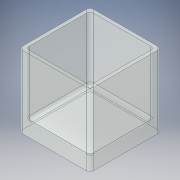
# Autodesk Inventor part: CandleHolder-3
Saved by Autodesk Inventor 2017 (Build 210142000, 142)
## iProperties
Created: 2016-10-20
Part Number: CandleHolder-3
Material: Glass
Document SubType Name: Modeling
Designer: Andrew Miyaguchi
Density: 2.18 g/cm^3
Appearance: Clear
Project: CandleHolder
Description: Glass Vase
Engineer: Andrew Miyaguchi
Author: andrew
Title: Glass Vase
Revision Number: 1
Autodesk Inventor part; units mm, degrees
ref_plane "YZ Plane" through (0, 0, 0) normal (1, 0, 0) x (0, 1, 0)
ref_plane "XZ Plane" through (0, 0, 0) normal (0, 1, 0) x (-1, 0, 0)
ref_plane "XY Plane" through (0, 0, 0) normal (0, 0, 1) x (1, 0, 0)
sketch "Sketch1" plane through (0, 0, 0) normal (0, 1, 0) x (-1, 0, 0)
  line L0 (-39.6875, 39.6875) -> (39.6875, 39.6875)
  line L1 (39.6875, 39.6875) -> (39.6875, -39.6875)
  line L2 (39.6875, -39.6875) -> (-39.6875, -39.6875)
  line L3 (-39.6875, -39.6875) -> (-39.6875, 39.6875)
  line L4 (-39.6875, 39.6875) -> (39.6875, -39.6875) construction
  line L5 (39.6875, 39.6875) -> (-39.6875, -39.6875) construction
  line L6 (-35.8775, 35.8775) -> (35.8775, 35.8775)
  line L7 (35.8775, 35.8775) -> (35.8775, -35.8775)
  line L8 (35.8775, -35.8775) -> (-35.8775, -35.8775)
  line L9 (-35.8775, -35.8775) -> (-35.8775, 35.8775)
  line L10 (-35.8775, 35.8775) -> (35.8775, -35.8775) construction
  line L11 (35.8775, 35.8775) -> (-35.8775, -35.8775) construction
  line L12 (0, -55.5625) -> (0, 55.5625) projected
  point P0 (0, 0)
  dimension "d0" = 3.81
  dimension "d10" = 79.375
  dimension "d11" = 45
  constraints: 24 end point, 4 midpoint, 4 parallel, 2 horizontal, 2 perpendicular, 1 point on line
  measures "d0" distance between parallel lines of L1 L7
  measures "d10" distance of L0.end L1.end
  measures "d11" angle of L12 L5
extrude "Extrusion1" add sketch "Sketch1" along normal blind 80.772 contours L0 L12 L6 L9 L8 L2 L3 | L0 L1 L2 L12 L8 L7 L6
extrude "Extrusion2" add sketch "Sketch1" along normal blind 9.652 contours L12 L8 L9 L6 | L6 L7 L8 L12
fillet "Fillet1" radius 3.81 12 edges at (-39.6875, 40.386, 39.6875) (-35.8775, 45.212, 35.8775) (-39.6875, 40.386, -39.6875) (-35.8775, 45.212, -35.8775) (35.8775, 45.212, -35.8775) (39.6875, 40.386, -39.6875) (35.8775, 45.212, 35.8775) (39.6875, 40.386, 39.6875) (-35.8775, 9.652, 0) (0, 9.652, 35.8775) (0, 9.652, -35.8775) (35.8775, 9.652, 0)
body "Solid1"
